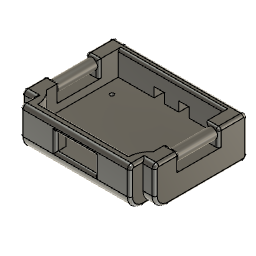
Carcasa Muñeca v11.5 (Autodesk Fusion 360 design; units mm, degrees)
Autodesk Fusion 360 part; units mm, degrees
sketch "Sketch10" plane through (0, 0, 0) normal (0, 0, 1) x (1, 0, 0)
  line L0 (0, -50) -> (0, 50) construction
  line L1 (0, 50) -> (-57, 50)
  line L2 (-57, 50) -> (-57, 0)
  line L3 (0, -50) -> (-45, -50)
  line L4 (-45, -50) -> (-45, -30)
  arc A0 (-57, 0) -> (-45, -30) centre (-7.0663, 2.5735) ccw
  line L5 (0, -50) -> (45, -50)
  line L6 (45, -50) -> (45, -30)
  arc A1 (45, -30) -> (57, 0) centre (7.0663, 2.5735) ccw
  line L7 (57, 50) -> (57, 0)
  line L8 (0, 50) -> (57, 50)
  dimension "d19" = 100
  dimension "d20" = 57
  dimension "d21" = 50
  dimension "d22" = 45
  dimension "d23" = 20
  dimension "d24" = 50
  dimension "d25" = 30
  constraint vertical L0
  constraint midpoint L0 origin
  constraint perpendicular L0 L1
  constraint perpendicular L1 L2
  constraint perpendicular L0 L3
  constraint perpendicular L3 L4
  constraint symmetric L3.start L0 L5.start
  constraint symmetric L1.start L0 L8.start
  constraint symmetric L0 L1.end L7.start
  constraint symmetric L0 L2.end A1.end
  constraint symmetric L0 L3.end L5.end
  constraint symmetric L0 L4.end L6.end
  constraint symmetric L0 A0 A1
  measures "d19" distance of L0.start L0.end
  measures "d20" distance of L0.end L1.end
  measures "d21" distance of L1.end L2.end
  measures "d22" distance of L0.start L3.end
  measures "d23" distance of L3.end L4.end
  measures "d24" radius of A0
  measures "d25" vertical distance of L2.end L4.end
sketch "Sketch12" plane through (0, 0, 0) normal (1, 0, 0) x (0, 1, 0)
  line L0 (0, 15.5) -> (0, -15.5) construction
  line L1 (0, 15.5) -> (40, 15.5)
  line L2 (43, 12.5) -> (43, -12.5)
  arc A0 (43, 12.5) -> (40, 15.5) centre (40, 12.5) ccw
  line L3 (0, 15.5) -> (-35, 15.5)
  line L4 (-38, 12.5) -> (-38, -5.5)
  arc A1 (-35, 15.5) -> (-38, 12.5) centre (-35, 12.5) ccw
  arc A2 (-38, -5.5) -> (-28, -15.5) centre (-28, -5.5) ccw
  arc A3 (40, -15.5) -> (43, -12.5) centre (40, -12.5) ccw
  line L5 (-28, -15.5) -> (40, -15.5)
  dimension "d30" = 3
  dimension "d34" = 3
  dimension "d35" = 10
  dimension "d36" = 18
  dimension "d38" = 3
  dimension "d40" = 25
  dimension "d308" = 35
  dimension "d309" = 40
  constraint vertical L0
  constraint midpoint L0 origin
  constraint perpendicular L0 L1
  constraint perpendicular L1 L2
  constraint tangent L1 A0
  constraint tangent L2 A0
  constraint perpendicular L0 L3
  constraint perpendicular L3 L4
  constraint tangent L4 A1
  constraint tangent L3 A1
  constraint tangent L4 A2
  constraint tangent L2 A3
  constraint tangent A3 L5
  measures "d30" radius of A0
  measures "d34" radius of A1
  measures "d35" radius of A2
  measures "d36" distance of L4.start L4.end
  measures "d38" radius of A3
  measures "d40" distance of L2.start L2.end
  measures "d308" distance of L0.start L3.end
  measures "d309" distance of L0.start L1.end
extrude "Extrude1" add sketch "Sketch12" along normal mid plane 84 makes body 1
ref_plane "PlanoDeObra18" through (-51, 2.5, 0) normal (-1, 0, 0) x (0, -1, 0)
sketch "Boceto31" plane through (-42, 0, 0) normal (-1, 0, 0) x (0, -1, 0)
  line L0 (35, 15.5) -> (-40, 15.5)
  line L1 (-43, 12.5) -> (-43, -12.5)
  arc A0 (-43, -12.5) -> (-40, -15.5) centre (-40, -12.5) ccw
  arc A1 (28, -15.5) -> (38, -5.5) centre (28, -5.5) ccw
  line L2 (38, -5.5) -> (38, 12.5)
  arc A2 (38, 12.5) -> (35, 15.5) centre (35, 12.5) ccw
  arc A3 (-43, -12.5) -> (-40, -15.5) centre (-40, -12.5) ccw
  line L3 (-40, -12.5) -> (-43, -12.5) construction
  line L4 (-40, -12.5) -> (-40, -15.5) construction
  line L5 (-40, -15.5) -> (18, -15.5)
  line L6 (-40, 15.5) -> (25, 15.5)
  line L7 (-43, 12.5) -> (-43, -12.5)
  arc A4 (28, 12.5) -> (24.9876, 15.5) centre (25, 12.5) ccw
  line L8 (25, 12.5) -> (28, 12.5) construction
  line L9 (25, 12.5) -> (24.9876, 15.5) construction
  arc A5 (18, -15.5) -> (28, -5.5) centre (18, -5.5) ccw
  line L10 (18, -5.5) -> (18, -15.5) construction
  line L11 (18, -5.5) -> (28, -5.5) construction
  line L12 (28, -5.5) -> (28, 12.5)
  line L13 (-40, -15.5) -> (28, -15.5)
  arc A6 (-40, 15.5) -> (-43, 12.4998) centre (-40, 12.5) ccw
  line L14 (-40, 12.5) -> (-40, 15.5) construction
  line L15 (-40, 12.5) -> (-43, 12.4998) construction
  dimension "d172" = 3
  dimension "d176" = 3
  dimension "d178" = 10
  dimension "d313" = 58
  dimension "d315" = 65
  dimension "d316" = 3
  dimension "d396" = 10
  constraint coincident A0.centre A3.centre
  constraint coincident A0.end A3.end
  constraint perpendicular L4 L5
  constraint parallel L0 L6
  constraint tangent A3 L7
  constraint tangent L6 A4
  constraint tangent L5 A5
  constraint tangent A5 L12
  constraint tangent A4 L12
  constraint perpendicular L6 L12
  constraint coincident L0.end L6.start
  constraint tangent L6 A6
  constraint tangent L7 A6
  measures "d172" radius of A3
  measures "d176" radius of A4
  measures "d178" radius of A5
  measures "d313" distance of A0.end L5.end
  measures "d315" distance of L0.end L6.end
  measures "d316" radius of A6
  measures "d396" distance of L2 L12
extrude "Extruir14" add sketch "Boceto31" along normal blind 9 contours L0 L1 A0 A3 L5 L6 L7 A4 A5 L12 L13 A6 bodies 1
sketch "Boceto32" plane through (42, 0, 0) normal (1, 0, 0) x (0, 1, 0)
  line L0 (40, 15.5) -> (-35, 15.5)
  arc A0 (-35, 15.5) -> (-38, 12.5) centre (-35, 12.5) ccw
  line L1 (-38, 12.5) -> (-38, -5.5)
  arc A1 (-38, -5.5) -> (-28, -15.5) centre (-28, -5.5) ccw
  arc A2 (40, -15.5) -> (43, -12.5) centre (40, -12.5) ccw
  line L2 (43, -12.5) -> (43, 12.5)
  arc A3 (43, 12.5) -> (40, 15.5) centre (40, 12.5) ccw
  arc A4 (43, 12.5) -> (40, 15.5) centre (40, 12.5) ccw
  line L3 (40, 12.5) -> (43, 12.5) construction
  line L4 (40, 12.5) -> (40, 15.5) construction
  line L5 (40, 15.5) -> (-25, 15.5)
  arc A5 (40, -15.5) -> (43, -12.5) centre (40, -12.5) ccw
  line L6 (40, -12.5) -> (40, -15.5) construction
  line L7 (40, -12.5) -> (43, -12.5) construction
  line L8 (-18, -15.526) -> (-18.0045, -5.526) construction
  arc A6 (-28.0045, -5.5235) -> (-18, -15.526) centre (-18.0045, -5.526) ccw
  line L9 (-18.0045, -5.526) -> (-28.0045, -5.5235) construction
  line L10 (-18.0045, -5.526) -> (-18, -15.526) construction
  arc A7 (-25, 15.5) -> (-28, 12.4949) centre (-25, 12.5) ccw
  line L11 (-25, 12.5) -> (-25, 15.5) construction
  line L12 (-25, 12.5) -> (-28, 12.4949) construction
  line L13 (-28, 12.4949) -> (-28.0045, -5.5235)
  line L14 (-18, -15.526) -> (40, -15.5)
  line L15 (-18, -15.526) -> (40, -15.5)
  line L16 (43, 12.5) -> (43, -12.5)
  dimension "d182" = 3
  dimension "d185" = 3
  dimension "d320" = 10
  dimension "d322" = 3
  dimension "d397" = 65
  dimension "d398" = 58
  constraint coincident A3.centre A4.centre
  constraint coincident L0.start A3.end
  constraint coincident A2.centre A5.centre
  constraint coincident A2.start A5.start
  constraint coincident L8.start A6.end
  constraint coincident L8.end A6.centre
  constraint tangent A6 L13
  constraint tangent L5 A7
  constraint tangent A6 L14
  constraint coincident L5.end A7.start
  constraint coincident L0 L5.end
  measures "d182" radius of A4
  measures "d185" radius of A5
  measures "d320" radius of A6
  measures "d322" radius of A7
  measures "d397" distance of L0.start L5.end
  measures "d398" distance of A2.start L8.start
extrude "Extruir15" add sketch "Boceto32" along normal blind 9 bodies 1
ref_plane "PlanoDeObra19" through (0, 2.5, -0.5) normal (0, 0, 1) x (0, -1, 0)
sketch "Boceto33" plane through (0, 0, -0.5) normal (0, 0, 1) x (1, 0, 0)
  line L0 (41, 36) -> (-41, 36)
  line L1 (-41, 36) -> (-41, -19)
  line L2 (41, -19) -> (41, 36)
  line L3 (-35, -30) -> (35, -30)
  line L4 (-51, 40) -> (-51, -18)
  line L5 (-42, 40) -> (51, 40)
  line L6 (-42, -35) -> (42, -35)
  line L7 (-42, -35) -> (-42, -25)
  line L8 (51, 40) -> (51, -25)
  arc A0 (-35, -30) -> (-41, -19) centre (-52.5597, -32.4416) ccw
  arc A1 (41, -19) -> (35, -30) centre (52.5597, -32.4416) ccw
  line L9 (42, -25) -> (42, -35)
  dimension "d257" = 10
  dimension "d310" = 4
  dimension "d325" = 70
  dimension "d327" = 55
  dimension "d330" = 10
  dimension "d399" = 7
  dimension "d400" = 7
  dimension "d415" = 5
  constraint horizontal L0
  constraint vertical L1
  constraint vertical L2
  constraint horizontal L3
  constraint equal L1 L2
  constraint equal A0 A1
  measures "d257" distance of L1 L4
  measures "d310" distance of L0 L5
  measures "d325" distance of L3.start L3.end
  measures "d327" distance of L0.end L1.end
  measures "d330" distance of L2 L8
  measures "d399" distance of L3.start L7
  measures "d400" distance of L3.end L9
  measures "d415" distance of L3 L6
extrude "Extruir16" cut sketch "Boceto33" along normal blind 16 and the other way blind 3 bodies 1
ref_plane "PlanoDeObra20" through (51, 7.5, 15.5) normal (-1, 0, 0) x (0, -1, 0)
sketch "Boceto34" plane through (51, 10, 10) normal (-1, 0, 0) x (0, 0, -1)
  line L0 (-5.5, 19) -> (7.5, 19)
  line L1 (7.5, 19) -> (7.5, -11)
  line L2 (7.5, -11) -> (-5.5, -11)
  line L3 (-5.5, -11) -> (-5.5, 19)
  line L4 (-5.5, -30) -> (-5.5, 35)
  dimension "d405" = 13
  dimension "d406" = 30
  dimension "d407" = 19
  constraint horizontal L0
  constraint vertical L1
  constraint horizontal L2
  constraint vertical L3
  constraint coincident L2.end L4
  measures "d405" distance of L1.end L2.end
  measures "d406" distance of L0.end L1.end
  measures "d407" distance of L2.end L4.start
extrude "Extruir17" cut sketch "Boceto34" along normal blind 15 bodies 1
ref_plane "PlanoDeObra21" through (46, -9, 9) normal (0, 1, 0) x (0, 0, -1)
sketch "Boceto35" plane through (46.5, -9, -6.0333) normal (0, 1, 0) x (1, 0, 0)
  circle A0 centre (-0.5, -16.5333) radius 4
  line L0 (4.5, -8.5333) -> (-5.5, -8.5333)
  line L1 (4.5, -8.5333) -> (4.5, -21.5333)
  line L2 (4.5, -21.5333) -> (-5.5, -21.5333)
  line L3 (-5.5, -21.5333) -> (-5.5, -8.5333)
  dimension "d210" = 8
  dimension "d408" = 5
  dimension "d409" = 8
  dimension "d418" = 5
  dimension "d419" = 5
  measures "d210" diameter of A0
  measures "d408" distance of A0.centre L2
  measures "d409" distance of A0.centre L0
  measures "d418" distance of A0.centre L3
  measures "d419" distance of A0.centre L1
extrude "Extruir18" add sketch "Boceto35" along normal up to surface (30 mm away) contours A0 bodies 1
sketch "Boceto43" plane through (-51, 0, 0) normal (-1, 0, 0) x (0, -1, 0)
  line L0 (28, -5.5) -> (28, 12.5)
  arc A0 (28, 12.5) -> (25, 15.5) centre (25, 12.5) ccw
  line L1 (25, 15.5) -> (-40, 15.5)
  arc A1 (-40, 15.5) -> (-43, 12.4998) centre (-40, 12.5) ccw
  line L2 (-43, 12.4998) -> (-43, -12.5)
  arc A2 (-43, -12.5) -> (-40, -15.5) centre (-40, -12.5) ccw
  line L3 (-40, -15.5) -> (18, -15.5)
  arc A3 (18, -15.5) -> (28, -5.5) centre (18, -5.5) ccw
  line L4 (-21, 2.5) -> (9, 2.5)
  line L5 (9, 2.5) -> (9, 15.5)
  line L6 (9, 15.5) -> (-21, 15.5)
  line L7 (-21, 15.5) -> (-21, 2.5)
  dimension "d361" = 13
  dimension "d411" = 19
  dimension "d412" = 30
  constraint horizontal L4
  constraint vertical L5
  constraint horizontal L6
  constraint vertical L7
  constraint coincident L5 L4.end
  constraint coincident L7.end L4
  constraint coincident L5.start L4
  constraint coincident L1 L6.end
  constraint coincident L7 L4.start
  measures "d361" distance of L4.start L6.end
  measures "d411" distance of L1.end L6.end
  measures "d412" distance of L4.end L4.start
extrude "Extruir26" cut sketch "Boceto43" against normal blind 15 contours L1 L4 L5 L6 L7 bodies 1
sketch "Boceto44" plane through (0, -9, 0) normal (0, 1, 0) x (-1, 0, 0)
  line L0 (51, 2.5) -> (51, 15.5)
  circle A0 centre (46, 10.5) radius 4
  line L1 (41, 2.5) -> (51, 2.5)
  line L2 (51, 15.5) -> (41, 15.5)
  line L3 (41, 2.5) -> (41, 15.5)
  dimension "d365" = 8
  dimension "d413" = 5
  dimension "d414" = 8
  dimension "d416" = 5
  dimension "d417" = 5
  measures "d365" diameter of A0
  measures "d413" distance of A0.centre L2
  measures "d414" distance of A0.centre L1
  measures "d416" distance of A0.centre L3
  measures "d417" distance of L0 A0.centre
extrude "Extruir27" add sketch "Boceto44" along normal up to surface (30 mm away) contours A0 bodies 1
ref_plane "PlanoDeObra22" through (-51, 7.5, 0) normal (-1, 0, 0) x (0, -1, 0)
ref_plane "PlanoDeObra23" through (0, 43, 0) normal (0, 1, 0) x (0, 0, 1)
ref_plane "PlanoDeObra25" through (0, -38, 3.5) normal (0, -1, 0) x (0, 0, -1)
sketch "Boceto36" plane through (0, -38, 3.5) normal (0, -1, 0) x (1, 0, 0)
  line L0 (-14.9998, 6) -> (15.0002, 6)
  line L1 (15.0002, 6) -> (15.0002, -7)
  line L2 (15.0002, -7) -> (-14.9998, -7)
  line L3 (-14.9998, -7) -> (-14.9998, 6)
  line L4 (-14.9998, 6) -> (15.0002, -7) construction
  line L5 (15.0002, 6) -> (-14.9998, -7) construction
  line L6 (-42, -9) -> (42, -9)
  line L7 (-42, 9) -> (42, 9)
  point P0 (0.0002, -0.5)
  dimension "d217" = 30
  dimension "d218" = 13
  dimension "d335" = 3
  constraint horizontal L0
  constraint perpendicular L0 L1
  constraint parallel L0 L2
  constraint parallel L1 L3
  constraint coincident L4 P0
  constraint coincident L5 P0
  measures "d217" distance of L1.end L2.end
  measures "d218" distance of L0.end L1.end
  measures "d335" distance of L0 L7
extrude "Extruir19" cut sketch "Boceto36" against normal blind 11 bodies 1
fillet "Empalme13" radius 2 9 edges at (-51, 43, -0.0001) (-51, 42.1213, -14.6213) (-51, 11, -15.5) (-51, -25.0711, -12.5711) (-51, -28, 3.5) (-51, -27.1213, 14.6213) (-51, -17, 15.5) (-51, 30.5, 15.5) (-51, 42.1214, 14.6212) on bodies 1
fillet "Empalme14" radius 2 5 edges at (-42, -23, -15.5) (-42, -35.0711, -12.5711) (-42, -38, 3.5) (-42, -37.1213, 14.6213) (-42, -30, 15.5) on bodies 1
fillet "Empalme15" radius 2 10 edges at (51, 11, -15.513) (51, 42.1213, -14.6213) (51, 43, 0) (51, 42.1213, 14.6213) (51, -17, 15.5) (51, 30.5, 15.5) (51, -27.1231, 14.6195) (51, -28.0022, 3.4857) (51, -25.0748, -12.5978) (51, 11, -15.513) on bodies 1
fillet "Empalme16" radius 2 5 edges at (42, -30, 15.5) (42, -37.1213, 14.6213) (42, -38, 3.5) (42, -35.0711, -12.5711) (42, -23.3625, -15.5) on bodies 1
sketch "Boceto39" plane through (0, 43, 0) normal (0, 1, 0) x (1, 0, 0)
  line L0 (49, 12.5771) -> (49, -12.4229)
  line L1 (13.5, 3.5) -> (5.5, 3.5)
  line L2 (5.5, 3.5) -> (5.5, -4)
  line L3 (5.5, -4) -> (13.5, -4)
  line L4 (13.5, -4) -> (13.5, 3.5)
  line L5 (-5.5, 3.5) -> (-13.5, 3.5)
  line L6 (-13.5, 3.5) -> (-13.5, -4)
  line L7 (-13.5, -4) -> (-5.5, -4)
  line L8 (-5.5, -4) -> (-5.5, 3.5)
  line L9 (-42, -12.5) -> (49, -12.5)
  line L10 (-49, -12.4998) -> (-49, 12.5)
  line L11 (49, 3.6424) -> (-49, 3.6424)
  line L12 (49, 12.5) -> (49, -12.5)
  dimension "d245" = 8
  dimension "d246" = 7.5
  dimension "d248" = 8
  dimension "d249" = 7.5
  dimension "d285" = 11
  dimension "d420" = 35.5
  dimension "d421" = 35.5
  constraint horizontal L1
  constraint vertical L2
  constraint horizontal L3
  constraint vertical L4
  constraint horizontal L5
  constraint vertical L6
  constraint horizontal L7
  constraint vertical L8
  constraint coincident L0 L11.start
  constraint coincident L10 L11.end
  constraint perpendicular L10 L11
  constraint coincident L11.start L12
  measures "d245" distance of L1.start L1.end
  measures "d246" distance of L1.start L3.end
  measures "d248" distance of L5.start L5.end
  measures "d249" distance of L5.start L7.end
  measures "d285" distance of L2 L8
  measures "d420" horizontal distance of L5.end L11.end
  measures "d421" horizontal distance of L1.start L11.start
extrude "Extruir22" cut sketch "Boceto39" against normal blind 8 bodies 1
sketch "Boceto40" plane through (0, 0, -3.5) normal (0, 0, 1) x (-1, 0, 0)
  line L0 (41, -36) -> (41, 19)
  line L1 (-41, 19) -> (-41, -36)
  line L2 (5.5, -43) -> (13.5, -43)
  line L3 (-41, -36) -> (-13.5, -36)
  line L4 (-13.5, -36) -> (-13.5, -43)
  line L5 (-5.5, -43) -> (-5.5, -36)
  line L6 (-5.5, -36) -> (5.5, -36)
  line L7 (5.5, -36) -> (5.5, -43)
  line L8 (13.5, -43) -> (13.5, -36)
  line L9 (13.5, -36) -> (41, -36)
  arc A0 (-41, 19) -> (-35, 30) centre (-52.5597, 32.4416) ccw
  arc A1 (35, 30) -> (41, 19) centre (52.5597, 32.4416) ccw
  line L10 (35, 30) -> (14.9998, 30)
  line L11 (14.9998, 30) -> (14.9998, 38)
  line L12 (14.9998, 38) -> (-15.0002, 38)
  line L13 (-15.0002, 38) -> (-15.0002, 30)
  line L14 (-15.0002, 30) -> (-35, 30)
  line L15 (-13.5, -43) -> (-5.5, -43)
sketch "Boceto41" plane through (0, 0, -3.5) normal (0, 0, 1) x (1, 0, 0)
  circle A0 centre (-31.95, 22.2) radius 1.55
  circle A1 centre (-31.95, -18) radius 1.55
  circle A2 centre (31.95, 22.2) radius 1.55
  circle A3 centre (31.95, -18) radius 1.55
  line L0 (31.95, -18) -> (-31.95, -18)
  line L1 (-31.95, -18) -> (-31.95, 22.2)
  line L2 (-31.95, 22.2) -> (31.95, 22.2)
  line L3 (31.95, 22.2) -> (31.95, -18)
  line L4 (-41, -19) -> (-41, 36)
  line L5 (41, 36) -> (41, -19)
  line L6 (-41, 36) -> (41, 36)
  line L7 (35, -30) -> (15.0002, -30)
  line L8 (-14.9998, -30) -> (-35, -30)
  dimension "d260" = 3.1
  dimension "d261" = 3.1
  dimension "d262" = 3.1
  dimension "d266" = 3.1
  dimension "d267" = 63.9
  dimension "d268" = 40.2
  dimension "d375" = 9.05
  dimension "d395" = 9.05
  dimension "d422" = 12
  constraint coincident A3.centre L0.start
  constraint coincident A1.centre L0.end
  constraint horizontal L0
  constraint coincident A0.centre L1.end
  constraint perpendicular L0 L1
  constraint coincident A2.centre L2.end
  measures "d260" diameter of A0
  measures "d261" diameter of A1
  measures "d262" diameter of A2
  measures "d266" diameter of A3
  measures "d267" distance of A1.centre A3.centre
  measures "d268" distance of A2.centre A3.centre
  measures "d375" distance of A0.centre L4
  measures "d395" distance of L3 L5
  measures "d422" distance of L0 L7
extrude "Extruir23" cut sketch "Boceto41" against normal blind 12 contours A0 L1 L2 | A0 L1 L2 | A2 L2 L3 | A2 L2 L3 | A1 L0 L1 | A1 L0 L1 | A3 L0 L3 | A3 L0 L3 bodies 1
fillet "Empalme21" radius 2 4 edges at (0.0002, -38, -3.5) (-14.9998, -38, 3) (0.0002, -38, 9.5) (15.0002, -38, 3) on bodies 1
fillet "Empalme24" radius 2 16 edges at (-51, 21, 8) (-50.4142, 21, 14.9142) (-45, 21, 15.5) (-41, 21, 9) (-41, -9, 9) (-45, -9, 15.5) (-50.4142, -9, 14.9142) (-51, -9, 8) (51, -9, 8) (50.4142, -9, 14.9142) (45, -9, 15.5) (41, -9, 9) (41, 21, 9) (45, 21, 15.5) (50.4142, 21, 14.9142) (51, 21, 8) on bodies 1
fillet "Empalme25" radius 2 1 edges at (0, 36, 15.5) on bodies 1
fillet "Empalme26" radius 2 1 edges at (0, -30, 15.5) on bodies 1
copy_body "Cuerpo - > Comp.3" bodies 1 removing the originals makes body 2 in component "Component'"
component "Component'" placed x (1, 0, 0) y (0, 1, 0) z (0, 0, 1) at (0, 0, 0)
